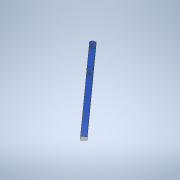
# Autodesk Inventor part: 零件2
Saved by Autodesk Inventor 2022 (Build 260153000, 153)
## iProperties
Created: 2023-03-09
Part Number: 零件2
Material: 一般
Document SubType Name: Modeling
Designer: JOU
Density: 1 g/cm^3
Appearance: 預設
Author: JOU
Autodesk Inventor part; units mm, degrees
ref_plane "YZ Plane" through (0, 0, 0) normal (1, 0, 0) x (0, 1, 0)
ref_plane "XZ Plane" through (0, 0, 0) normal (0, 1, 0) x (-1, 0, 0)
ref_plane "XY Plane" through (0, 0, 0) normal (0, 0, 1) x (1, 0, 0)
sketch "草圖1" plane through (0, 0, 0) normal (0, 1, 0) x (-1, 0, 0)
  line L0 (0, 0) -> (14.7102, 0)
  line L1 (14.7102, 0) -> (14.7102, -16.4216)
  line L2 (14.7102, -16.4216) -> (0, 0)
  constraints: 6 end point, 1 horizontal, 1 perpendicular
extrude "擠出1" add sketch "草圖1" along normal blind 1
sketch "草圖2" plane through (0, 1, 0) normal (0, 1, 0) x (1, 0, 0)
  circle A0 centre (-13.9602, 14.4603) radius 0.75
  line L0 (-14.7102, 16.4216) -> (-14.7102, 0) projected
  line L1 (0, 0) -> (-14.7102, 16.4216) projected
  dimension "d2" = 1.5
  constraints: 2 tangent, 1 centre point
  measures "d2" diameter of A0
extrude "擠出2" add sketch "草圖2" along normal blind 1 contours A0
sketch "草圖4" plane through (0, 1, 0) normal (0, 1, 0) x (1, 0, 0)
  line L0 (-14.7102, 0) -> (0, 0) projected
  line L1 (-2.0138, 0) -> (-14.7102, 14.1735)
  line L2 (0, 0) -> (-13.4016, 14.9607) projected
  line L3 (-14.7102, 14.4603) -> (-14.7102, 0) projected
  point P0 (-1.1201, 1.2504)
  dimension "d7" = 1.5
  constraints: 2 end point, 2 point on line, 1 parallel
  measures "d7" distance between parallel lines of L2 L1
extrude "擠出4" cut sketch "草圖4" against normal blind 10
sketch "草圖5" plane through (0, 1, 0) normal (0, 1, 0) x (1, 0, 0)
  circle A0 centre (-6.9543, 6.6393) radius 0.75
  line L0 (-14.5188, 13.9599) -> (-2.0138, 0) projected
  line L1 (0, 0) -> (-13.4016, 14.9607) projected
  circle A1 centre (-13.9602, 14.4603) radius 0.75 projected
  dimension "d11" = 10.5
  constraints: 2 tangent, 1 centre point
  measures "d11" distance of A1.centre A0.centre
extrude "擠出5" add sketch "草圖5" along normal up to surface (1 mm away) contours A0
sketch "草圖6" plane through (0, 1, 0) normal (0, 1, 0) x (1, 0, 0)
  line L0 (-7.513, 6.1389) -> (-2.0138, 0) projected
  line L1 (0, 0) -> (-6.3957, 7.1398) projected
  line L2 (-2.0138, 0) -> (-0.8965, 1.0008)
  line L3 (-0.8965, 1.0008) -> (10.5719, -11.8019)
  line L4 (10.5719, -11.8019) -> (9.4546, -12.8027)
  line L5 (9.4546, -12.8027) -> (-2.0138, 0)
  constraints: 8 end point, 2 parallel, 1 perpendicular, 1 point on line
extrude "擠出6" add sketch "草圖6" against normal up to surface (1 mm away)
